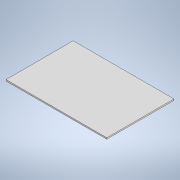
# Autodesk Inventor part: placa pcb 100x150mm
Saved by Autodesk Inventor 2020 (Build 240168000, 168)
## iProperties
Created: 2020-05-31
Part Number: placa pcb 100x150mm
Material: Genérico
Document SubType Name: Modeling
Designer: Pipi
Density: 1 g/cm^3
Appearance: Valor por defecto
Author: Pipi
Autodesk Inventor part; units mm, degrees
ref_plane "YZ Plane" through (0, 0, 0) normal (1, 0, 0) x (0, 1, 0)
ref_plane "XZ Plane" through (0, 0, 0) normal (0, 1, 0) x (-1, 0, 0)
ref_plane "XY Plane" through (0, 0, 0) normal (0, 0, 1) x (1, 0, 0)
sketch "Boceto1" plane through (0, 0, 0) normal (0, 1, 0) x (-1, 0, 0)
  line L0 (8.0294, 11.328) -> (8.0294, -88.672)
  line L1 (8.0294, -88.672) -> (-141.9706, -88.672)
  line L2 (-141.9706, -88.672) -> (-141.9706, 11.328)
  line L3 (-141.9706, 11.328) -> (8.0294, 11.328)
  point P0 (0, 0)
  dimension "d0" = 100
  dimension "d1" = 150
  constraints: 8 end point, 3 perpendicular, 1 vertical
  measures "d0" distance of L0.start L0.end
  measures "d1" distance of L0.end L1.end
extrude "Extrusión1" add sketch "Boceto1" along normal blind 2
